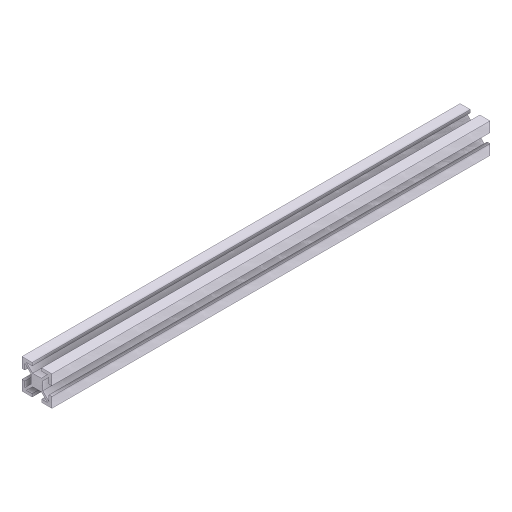
# Autodesk Inventor part: front axle
Saved by Autodesk Inventor 2023 (Build 270158000, 158)
## iProperties
Created: 2023-03-28
Part Number: front axle
Material: Generic
Document SubType Name: Modeling
Designer: Juyoung Han
Density: 1 g/cm^3
Appearance: Weld - Aluminum
Author: Juyoung Han
Autodesk Inventor part; units mm, degrees
ref_plane "YZ Plane" through (0, 0, 0) normal (1, 0, 0) x (0, 1, 0)
ref_plane "XZ Plane" through (0, 0, 0) normal (0, 1, 0) x (-1, 0, 0)
ref_plane "XY Plane" through (0, 0, 0) normal (0, 0, 1) x (1, 0, 0)
sketch "Sketch1" plane through (0, 0, 0) normal (0, 0, 1) x (1, 0, 0)
  line L0 (-2.9393, 4) -> (2.9393, 4)
  line L1 (4, 2.9393) -> (4, -2.9393)
  line L2 (2.9393, -4) -> (-2.9393, -4)
  line L3 (-4, -2.9393) -> (-4, 2.9393)
  line L4 (0, 0) -> (4, -4) construction
  line L5 (-0.5303, -0.5303) -> (-4, -4) construction
  line L6 (5.0607, 4) -> (10, 4) construction
  line L7 (8.2426, 7.182) -> (8.2426, 3.2426)
  line L8 (8.2426, 3.2426) -> (10.2426, 3.2426)
  line L9 (10.2426, 3.2426) -> (10.2426, 10.2426)
  line L10 (10.2426, 10.2426) -> (3.2426, 10.2426)
  line L11 (3.2426, 10.2426) -> (3.2426, 8.2426)
  line L12 (3.2426, 8.2426) -> (7.182, 8.2426)
  line L13 (2.9393, 4) -> (7.182, 8.2426)
  line L14 (4, 2.9393) -> (8.2426, 7.182)
  line L15 (-8.2426, 7.182) -> (-8.2426, 3.2426)
  line L16 (-8.2426, 3.2426) -> (-10.2426, 3.2426)
  line L17 (-10.2426, 3.2426) -> (-10.2426, 10.2426)
  line L18 (-10.2426, 10.2426) -> (-3.2426, 10.2426)
  line L19 (-3.2426, 10.2426) -> (-3.2426, 8.2426)
  line L20 (-3.2426, 8.2426) -> (-7.182, 8.2426)
  line L21 (-2.9393, 4) -> (-7.182, 8.2426)
  line L22 (-4, 2.9393) -> (-8.2426, 7.182)
  line L23 (-2.9393, -4) -> (2.9393, -4)
  line L24 (4, -2.9393) -> (4, 2.9393)
  line L25 (-4, 2.9393) -> (-4, -2.9393)
  line L26 (-4, -4) -> (0, 0) construction
  line L27 (5.0607, -4) -> (10, -4) construction
  line L28 (8.2426, -7.182) -> (8.2426, -3.2426)
  line L29 (8.2426, -3.2426) -> (10.2426, -3.2426)
  line L30 (10.2426, -3.2426) -> (10.2426, -10.2426)
  line L31 (10.2426, -10.2426) -> (3.2426, -10.2426)
  line L32 (3.2426, -10.2426) -> (3.2426, -8.2426)
  line L33 (3.2426, -8.2426) -> (7.182, -8.2426)
  line L34 (2.9393, -4) -> (7.182, -8.2426)
  line L35 (4, -2.9393) -> (8.2426, -7.182)
  line L36 (-3.2426, -10.2426) -> (-3.2426, -8.2426)
  line L37 (-2.9393, -4) -> (-7.182, -8.2426)
  line L38 (-8.2426, -7.182) -> (-8.2426, -3.2426)
  line L39 (-3.2426, -8.2426) -> (-7.182, -8.2426)
  line L40 (-4, -2.9393) -> (-8.2426, -7.182)
  line L41 (-10.2426, -3.2426) -> (-10.2426, -10.2426)
  line L42 (-10.2426, -10.2426) -> (-3.2426, -10.2426)
  line L43 (-8.2426, -3.2426) -> (-10.2426, -3.2426)
  point P0 (0, 0)
  point P1 (-4, 4)
  point P2 (-4, 4)
  dimension "d0" = 8
  constraints: 88 end point, 5 point on line, 4 perpendicular, 3 parallel, 2 horizontal, 1 vertical
  measures "d0" distance of L4.end L5.end
extrude "Extrusion1" add sketch "Sketch1" along normal mid plane 300
body "Solid1"
